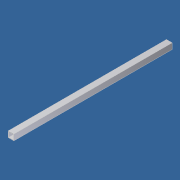
# Autodesk Inventor part: GE-11041-03
Saved by Autodesk Inventor 2012 (Build 160160000, 160)
## iProperties
Created: 2010-09-30
Part Number: GE-11041-03
Document SubType Name: Modeling
Designer: mcyr
Density: 1 g/cm^3
Description: Top & Bottom Braces
Material: Default
Title: Top & Bottom Braces
Author: mcyr
Autodesk Inventor part; units mm, degrees
ref_plane "YZ Plane" through (0, 0, 0) normal (1, 0, 0) x (0, 1, 0)
ref_plane "XZ Plane" through (0, 0, 0) normal (0, 1, 0) x (-1, 0, 0)
ref_plane "XY Plane" through (0, 0, 0) normal (0, 0, 1) x (1, 0, 0)
sketch "Sketch1" plane through (0, 0, 0) normal (0, 0, 1) x (1, 0, 0)
  line L0 (-25.4098, 25.5063) -> (19.0402, 25.5063)
  line L1 (19.0402, 25.5063) -> (19.0402, -18.9437)
  line L2 (19.0402, -18.9437) -> (-25.4098, -18.9437)
  line L3 (-25.4098, -18.9437) -> (-25.4098, 25.5063)
  line L4 (15.8652, 22.3313) -> (-22.2348, 22.3313)
  line L5 (-22.2348, 22.3313) -> (-22.2348, -15.7687)
  line L6 (-22.2348, -15.7687) -> (15.8652, -15.7687)
  line L7 (15.8652, -15.7687) -> (15.8652, 22.3313)
  point P0 (0, 0)
  dimension "d0" = 44.45
  dimension "d1" = 44.45
  dimension "d2" = 3.175
  constraints: 16 end point, 4 parallel, 2 perpendicular, 1 horizontal, 3 other
  measures "d0" distance of L0.start L0.end
  measures "d1" distance of L2.end L0.start
  measures "d2" distance between parallel lines of L0 L4
extrude "Extrusion1" add sketch "Sketch1" along normal blind 1219.2
body "Solid1"
